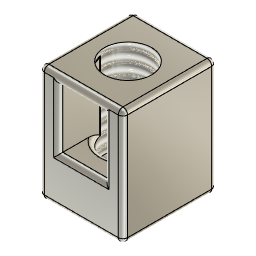
RENOGY SOLAR CHARGE CONTROLLER v14 (Autodesk Fusion 360 archive; units mm, degrees)
design "ScrewMount"
Autodesk Fusion 360 part; units mm, degrees
note: some values were not read from the file. Chosen so that the rebuilt part matches the saved one: which face or edge a step refers to.
sketch "Sketch1" plane through (0, 0, 0) normal (0, 0, 1) x (1, 0, 0)
  line L0 (0, 0) -> (4.572, 0)
  line L1 (4.572, 0) -> (4.572, 5.1308)
  line L2 (4.572, 5.1308) -> (0, 5.1308)
  line L3 (0, 5.1308) -> (0, 0)
  dimension "d1" = 5.1308
  dimension "d2" = 4.572
  constraint horizontal L0
  constraint vertical L1
  constraint horizontal L2
  constraint vertical L3
  constraint coincident L0.start L3.end
  measures "d1" distance of L0.start L2.end
  measures "d2" distance of L0.start L0.end
extrude "Extrude1" add sketch "Sketch1" along normal blind 6.35
sketch "Sketch2" plane through (0, 0, 6.35) normal (0, 0, 1) x (-1, 0, 0)
  line L0 (0, -5.1308) -> (0, 0)
  line L1 (0, 0) -> (-4.572, 0)
  line L2 (-4.572, 0) -> (-4.572, -5.1308)
  line L3 (-4.572, -5.1308) -> (0, -5.1308)
  line L4 (0, -5.1308) -> (-4.572, 0) construction
  line L5 (-4.572, -5.1308) -> (0, 0) construction
  circle A0 centre (-2.286, -2.5654) radius 1.27
  dimension "d5" = 2.54
  constraint coincident L0.start L3.end
  constraint coincident L1.end L2.start
  constraint coincident L2.end L3.start
  constraint coincident L0.end L1.start
  constraint midpoint L4 A0.centre
  measures "d5" diameter of A0
hole "Hole1" at (2.286, 2.5654, 6.35) direction (0, 0, -1) diameter 2.5908 depth 5.08 tip angle 118
thread "Thread1" "ANSI Unified Screw Threads 0.125(#5) 5-40 UNC 2B"
sketch "Sketch3" plane through (0, 0, 0) normal (0, -1, 0) x (1, 0, 0)
  line L0 (0, 0) -> (4.572, 0)
  line L1 (4.572, 0) -> (4.572, 6.35)
  line L2 (4.572, 6.35) -> (0, 6.35)
  line L3 (0, 6.35) -> (0, 0)
  line L4 (1.016, 5.842) -> (3.556, 5.842)
  line L5 (3.556, 5.842) -> (3.556, 2.54)
  line L6 (3.556, 2.54) -> (1.016, 2.54)
  line L7 (1.016, 2.54) -> (1.016, 5.842)
  line L8 (0, 6.35) -> (1.016, 5.842)
  line L9 (4.572, 6.35) -> (3.556, 5.842)
  line L10 (3.556, 2.54) -> (4.572, 0)
  line L11 (1.016, 2.54) -> (0, 0)
  dimension "d9" = 2.54
  dimension "d10" = 0.508
  dimension "d11" = 2.54
  constraint horizontal L4
  constraint vertical L5
  constraint horizontal L6
  constraint vertical L7
  constraint coincident L2.end L3.start
  constraint coincident L1.end L2.start
  constraint coincident L0.end L1.start
  constraint coincident L0.start L3.end
  constraint equal L8 L9
  measures "d9" distance of L4.start L4.end
  measures "d10" distance of L2 L4
  measures "d11" distance of L0 L6
extrude "Extrude2" cut sketch "Sketch3" against normal blind 2.54 contours L4 L5 L6 L7
fillet "Fillet1" radius 0.254 12 edges at (2.286, 0, 6.35) (4.572, 2.5654, 6.35) (4.572, 0, 3.175) (0, 0, 3.175) (0, 2.5654, 6.35) (0, 5.1308, 3.175) (2.286, 5.1308, 6.35) (2.286, 0, 0) (4.572, 2.5654, 0) (0, 2.5654, 0) (4.572, 5.1308, 3.175) (2.286, 5.1308, 0)
fillet "Fillet2" radius 0.254 8 edges at (1.016, 0, 4.191) (2.286, 0, 5.842) (3.556, 0, 4.191) (2.286, 0, 2.54) (3.1068, 1.5632, 5.842) (1.4652, 1.5632, 5.842) (1.4652, 1.5632, 2.54) (3.1068, 1.5632, 2.54)
